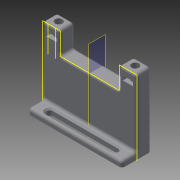
# Autodesk Inventor part: soporte
Saved by Autodesk Inventor 2015 SP1 (Build 190203100, 203)
## iProperties
Created: 2015-06-12
Part Number: soporte
Material: Generic
Document SubType Name: Modeling
Designer: pc
Density: 1 g/cm^3
Appearance: Default
Author: pc
Autodesk Inventor part; units mm, degrees
ref_plane "YZ Plane" through (0, 0, 0) normal (1, 0, 0) x (0, 1, 0)
ref_plane "XZ Plane" through (0, 0, 0) normal (0, 1, 0) x (-1, 0, 0)
ref_plane "XY Plane" through (0, 0, 0) normal (0, 0, 1) x (1, 0, 0)
sketch "Sketch1" plane through (0, 0, 0) normal (0, 0, 1) x (1, 0, 0)
  line L0 (-64, 10) -> (0, 10)
  line L1 (0, 10) -> (0, 0)
  line L2 (0, 0) -> (-64, 0)
  line L3 (-64, 0) -> (-64, 10)
  dimension "d0" = 64
  dimension "d1" = 10
  constraints: 8 end point, 2 parallel, 1 coincident, 1 horizontal, 1 perpendicular
  measures "d0" distance of L1.end L2.end
  measures "d1" distance of L2.end L0.start
extrude "Extrusion1" add sketch "Sketch1" along normal blind 50
sketch "Sketch2" plane through (0, 0, 50) normal (0, 0, 1) x (1, 0, 0)
  line L0 (0, 10) -> (-64, 10) projected
  line L1 (-64, 10) -> (-64, 0) projected
  line L2 (-64, 0) -> (0, 0) projected
  line L3 (0, 0) -> (0, 10) projected
  circle A0 centre (-58, 5) radius 2.5
  circle A1 centre (-6, 5) radius 2.5
  line L4 (-32, 17) -> (-32, -12)
  line L5 (-64, 10) -> (-64, 0) projected
  line L6 (-64, 5) -> (0, 5)
  dimension "d4" = 52
  dimension "d5" = 5
  dimension "d6" = 32
  constraints: 4 end point, 2 centre point, 2 midpoint, 1 equal radius, 1 point on line, 1 symmetric about line, 1 vertical
  measures "d4" distance of A1.centre A0.centre
  measures "d5" diameter of A0
  measures "d6" distance between parallel lines of L4 L1
extrude "Extrusion2" cut sketch "Sketch2" against normal blind 18 contours L6 A1 | A1 L6 | L6 A0 | A0 L6
sketch "Sketch3" plane through (0, 0, 50) normal (0, 0, 1) x (1, 0, 0)
  circle A0 centre (-6, 5) radius 2.5 projected
  circle A1 centre (-58, 5) radius 2.5 projected
  line L0 (0, 10) -> (-64, 10) projected
  line L1 (-64, 10) -> (-64, 0) projected
  line L2 (-64, 0) -> (0, 0) projected
  line L3 (0, 0) -> (0, 10) projected
  line L4 (-64, 0) -> (0, 0) projected
  line L5 (-52, 10) -> (-12, 10)
  line L6 (-12, 10) -> (-12, 0)
  line L7 (-12, 0) -> (-52, 0)
  line L8 (-52, 0) -> (-52, 10)
  dimension "d9" = 12
  dimension "d10" = 12
  constraints: 8 end point, 2 parallel, 2 point on line, 1 horizontal, 1 perpendicular
  measures "d9" distance between parallel lines of L8 L1
  measures "d10" distance between parallel lines of L3 L6
ref_plane "Work Plane1" through (-32, 0, 0) normal (-1, 0, 0) x (0, 0, 1)
extrude "Extrusion3" cut sketch "Sketch3" against normal blind 15 contours L6 L2 L8 L0
sketch "Sketch4" plane through (-64, 0, 0) normal (0, -1, 0) x (1, 0, 0)
  line L0 (12, 35) -> (12, 50) projected
  line L1 (0, 50) -> (12, 50) projected
  line L2 (0, 0) -> (0, 50) projected
  line L3 (64, 0) -> (0, 0) projected
  line L4 (64, 0) -> (64, 50) projected
  line L5 (52, 50) -> (64, 50) projected
  line L6 (52, 50) -> (52, 35) projected
  line L7 (52, 35) -> (12, 35) projected
  line L8 (8.5, 50) -> (8.5, 32) projected
  line L9 (3.5, 50) -> (3.5, 32) projected
sketch "Sketch5" plane through (-64, 0, 0) normal (0, -1, 0) x (1, 0, 0)
  line L0 (2.5, 45) -> (9.5, 45)
  line L1 (9.5, 45) -> (9.5, 42)
  line L2 (9.5, 42) -> (2.5, 42)
  line L3 (2.5, 42) -> (2.5, 45)
  line L4 (3.5, 50) -> (8.5, 50) projected
  line L5 (6, 50) -> (6, 38)
  line L6 (0, 50) -> (12, 50) projected
  point P0 (64, 0)
  dimension "d13" = 7
  dimension "d14" = 3
  dimension "d15" = 5
  constraints: 10 end point, 3 midpoint, 2 parallel, 1 horizontal, 1 perpendicular, 1 symmetric about line
  measures "d13" distance of L1.end L2.end
  measures "d14" distance of L0.end L1.end
  measures "d15" distance between parallel lines of L0 L4
extrude "Extrusion4" cut sketch "Sketch5" against normal blind 8.5
mirror "Mirror1" about plane through (-32, 0, 0) normal (-1, 0, 0) of "Extrusion4"
sketch "Sketch6" plane through (0, 0, 0) normal (0, 0, -1) x (-1, 0, 0)
  line L0 (64, 10) -> (0, 10) projected
  line L1 (0, 10) -> (0, 0) projected
  line L2 (0, 0) -> (64, 0) projected
  line L3 (64, 0) -> (64, 10) projected
  line L4 (0, 0) -> (64, 0)
  line L5 (64, 0) -> (64, -10)
  line L6 (64, -10) -> (0, -10)
  line L7 (0, -10) -> (0, 0)
  dimension "d30" = 10
  constraints: 8 end point, 2 parallel, 1 horizontal, 1 perpendicular
  measures "d30" distance of L2.end L5.end
extrude "Extrusion5" add sketch "Sketch6" against normal blind 4 contours L5 L6 L7 L2
sketch "Sketch7" plane through (0, 0, 4) normal (0, 0, 1) x (1, 0, 0)
  line L0 (0, -10) -> (0, 0) projected
  line L1 (-64, 0) -> (0, 0) projected
  line L2 (-64, 0) -> (-64, -10) projected
  line L3 (-64, -10) -> (0, -10) projected
  line L4 (-54, -5) -> (-10, -5) construction
  line L5 (-54, -7.25) -> (-10, -7.25)
  line L6 (-10, -2.75) -> (-54, -2.75)
  arc A0 (-54, -2.75) -> (-54, -7.25) centre (-54, -5) ccw
  arc A1 (-10, -7.25) -> (-10, -2.75) centre (-10, -5) ccw
  point P0 (-32, -5)
  dimension "d20" = 4.5
  dimension "d22" = 10
  dimension "d23" = 10
  dimension "d24" = 5
  constraints: 8 end point, 4 point on circle, 4 tangent, 2 centre point, 1 horizontal, 1 midpoint, 1 parallel
  measures "d20" diameter of A1
  measures "d22" distance from line of L2 L4.start
  measures "d23" distance from line of L0 L4.end
  measures "d24" distance from line of L1 point (-32, -5)
extrude "Extrusion6" cut sketch "Sketch7" against normal through all contours A0 L6 A1 L5
chamfer "Chamfer1" distance 1 angle 45 4 edges at (-32, -2.75, 4) (-7.75, -5, 4) (-32, -7.25, 4) (-56.25, -5, 4)
fillet "Fillet1" radius 2 26 edges at (-64, 10, 25) (-52, 10, 42.5) (-58, 10, 50) (-52, 5, 50) (-64, 5, 50) (-64, 0, 27) (-32, 10, 35) (-12, 10, 42.5) (-12, 5, 50) (-6, 10, 50) (0, 5, 50) (0, 10, 25) (-12, 5, 35) (-32, 0, 35) (-52, 5, 35) (-58, 0, 50) (-52, 0, 42.5) (-12, 0, 42.5) (-32, 0, 4) (0, -5, 4) (-32, -10, 4) (-64, -5, 4) (-64, -10, 2) (0, -10, 2) (-6, 0, 50) (0, 0, 27)
body "Solid1"
